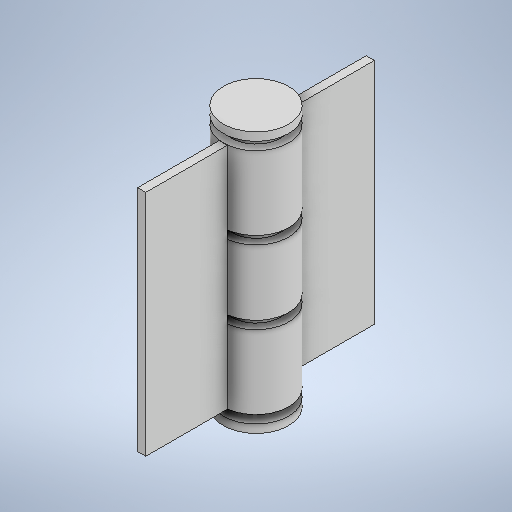
# Autodesk Inventor part: Schanier 1.0
Saved by Autodesk Inventor 2025.2 (Build 292293000, 293)
## iProperties
Created: 2024-11-18
Part Number: Schanier 1.0
Material: Generic
Document SubType Name: Modeling
Designer: jurre
Density: 1 g/cm^3
Appearance: Default
Author: jurre
Autodesk Inventor part; units mm, degrees
ref_plane "YZ Plane" through (0, 0, 0) normal (1, 0, 0) x (0, 1, 0)
ref_plane "XZ Plane" through (0, 0, 0) normal (0, 1, 0) x (-1, 0, 0)
ref_plane "XY Plane" through (0, 0, 0) normal (0, 0, 1) x (1, 0, 0)
sketch "Sketch1" plane through (0, 0, 0) normal (0, 1, 0) x (-1, 0, 0)
  circle A0 centre (0, 0) radius 2.5
  circle A1 centre (0, 0) radius 3
  circle A2 centre (0, 0) radius 4
  dimension "d0" = 5
  dimension "d1" = 6
  dimension "d2" = 8
  constraints: 3 centre point, 3 coincident
  measures "d0" diameter of A0
  measures "d1" diameter of A1
  measures "d2" diameter of A2
extrude "Extrusion1" add sketch "Sketch1" along normal blind 1 contours A0 | A1 | A2
extrude "Extrusion2" add sketch "Sketch1" along normal blind 30 from surface at 1 contours A0
extrude "Extrusion3" add sketch "Sketch1" along normal blind 1 from surface at 31 contours A0 | A1 | A2
sketch "Sketch2" plane through (0, 32, 0) normal (0, 1, 0) x (1, 0, 0)
  circle A0 centre (0, 0) radius 4
  circle A1 centre (0, 0) radius 3
  dimension "d9" = 8
  dimension "d10" = 6
  constraints: 2 centre point, 2 coincident
  measures "d9" diameter of A0
  measures "d10" diameter of A1
extrude "Extrusion4" add sketch "Sketch2" along normal blind 9 separate body
move or copy body "Move Body1" bodies to move or copy 2 copy no translate (0, -10, 0)
extrude "Extrusion5" add sketch "Sketch2" along normal blind 8 separate body
extrude "Extrusion6" add sketch "Sketch2" along normal blind 9 separate body
move or copy body "Move Body2" bodies to move or copy 2 copy no translate (0, -1, 0)
move or copy body "Move Body3" bodies to move or copy 4 copy no translate (0, -30, 0)
move or copy body "Move Body4" bodies to move or copy 3 copy no translate (0, -20, 0)
combine bodies "Combine1" operation type add bodies to combine 2 4
sketch "Sketch3" plane through (0, 0, 0) normal (1, 0, 0) x (0, 1, 0)
  line L0 (2, -4) -> (2, 4) projected
  line L1 (2, 4) -> (30, 4)
  line L2 (30, 4) -> (30, 14)
  line L3 (30, 14) -> (2, 14)
  line L4 (2, 14) -> (2, 4)
  point P0 (0, 0)
  dimension "d29" = 10
  dimension "d30" = 28
  constraints: 8 end point, 2 parallel, 1 horizontal, 1 perpendicular
  measures "d29" distance of L1.end L2.end
  measures "d30" distance of L2.end L3.end
extrude "Extrusion7" add sketch "Sketch3" along normal mid plane 1 separate body
combine bodies "Combine2" operation type add bodies to combine 2 5
sketch "Sketch4" plane through (0, 0, 0) normal (1, 0, 0) x (0, 1, 0)
  line L0 (30, -4) -> (30, 4) projected
  line L1 (30, -4) -> (2, -4)
  line L2 (2, -4) -> (2, -14)
  line L3 (2, -14) -> (30, -14)
  line L4 (30, -14) -> (30, -4)
  point P0 (0, 0)
  dimension "d33" = 10
  dimension "d34" = 28
  constraints: 8 end point, 2 parallel, 1 horizontal, 1 perpendicular
  measures "d33" distance of L3.end L0.start
  measures "d34" distance of L2.end L3.end
extrude "Extrusion8" add sketch "Sketch4" along normal mid plane 1 separate body
combine bodies "Combine3" operation type add bodies to combine 3 6
body "Solid1"
body "Solid2"
body "Solid3"
